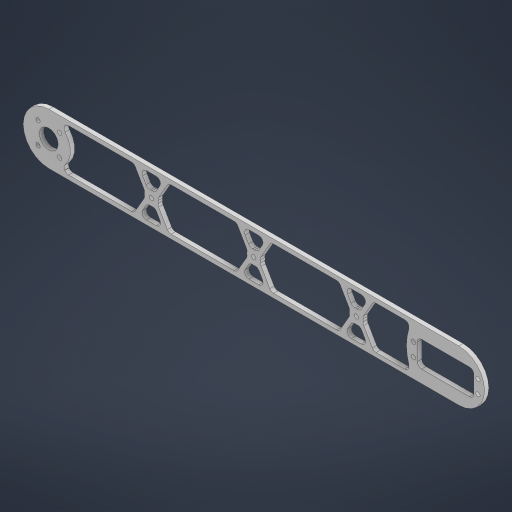
# Autodesk Inventor part: Arm2ndLink
Saved by Autodesk Inventor 2023 (Build 270158000, 158)
## iProperties
Created: 2023-12-24
Part Number: Arm2ndLink
Material: Generic
Document SubType Name: Modeling
Designer: kelle
Density: 1 g/cm^3
Appearance: Default
Author: kelle
Autodesk Inventor part; units mm, degrees
ref_plane "YZ Plane" through (0, 0, 0) normal (1, 0, 0) x (0, 1, 0)
ref_plane "XZ Plane" through (0, 0, 0) normal (0, 1, 0) x (-1, 0, 0)
ref_plane "XY Plane" through (0, 0, 0) normal (0, 0, 1) x (1, 0, 0)
sketch "Sketch1" plane through (0, 0, 0) normal (0, 0, 1) x (1, 0, 0)
  line L0 (152.4, 0) -> (-152.4, 0) construction
  line L1 (152.4, 19.05) -> (-152.4, 19.05)
  line L2 (-152.4, -19.05) -> (152.4, -19.05)
  arc A0 (152.4, -19.05) -> (152.4, 19.05) centre (152.4, 0) ccw
  arc A1 (-152.4, 19.05) -> (-152.4, -19.05) centre (-152.4, 0) ccw
  circle A2 centre (-152.4, 0) radius 7
  line L3 (-160.4, -8) -> (-144.4, -8) construction
  line L4 (-144.4, -8) -> (-144.4, 8) construction
  line L5 (-144.4, 8) -> (-160.4, 8) construction
  line L6 (-160.4, 8) -> (-160.4, -8) construction
  line L7 (-160.4, -8) -> (-144.4, 8) construction
  line L8 (-144.4, -8) -> (-160.4, 8) construction
  circle A3 centre (-160.4, 8) radius 1.5875
  circle A4 centre (-144.4, 8) radius 1.5875
  circle A5 centre (-160.4, -8) radius 1.5875
  circle A6 centre (-144.4, -8) radius 1.5875
  circle A7 centre (0, 0) radius 2
  circle A8 centre (-76.2, 0) radius 2
  circle A9 centre (76.2, 0) radius 2
  circle A10 centre (0, 0) radius 2
  circle A11 centre (152.4, 0) radius 3
  line L9 (152.4, 0) -> (166.6, 0) construction
  line L10 (166.6, 0) -> (166.6, 4.95) construction
  circle A12 centre (166.6, 4.95) radius 1.5875
  circle A13 centre (118.6, 4.95) radius 1.5875
  circle A14 centre (166.6, -4.95) radius 1.5875
  circle A15 centre (118.6, -4.95) radius 1.5875
  line L11 (166.6, 4.95) -> (163.6, 4.95) construction
  line L12 (163.6, 9.525) -> (121.6, 9.525)
  line L13 (121.6, 9.525) -> (121.6, -9.525)
  line L14 (163.6, -9.525) -> (163.6, 9.525)
  line L15 (121.6, -9.525) -> (163.6, -9.525)
  dimension "d0" = 152.4
  dimension "d1" = 38.1
  dimension "d2" = 14
  dimension "d3" = 16
  dimension "d4" = 16
  dimension "d5" = 3.175
  dimension "d8" = 16
  dimension "d11" = 16
  dimension "d14" = 4
  dimension "d17" = 76.2
  dimension "d20" = 76.2
  dimension "d23" = 6
  dimension "d24" = 14.2
  dimension "d25" = 4.95
  dimension "d27" = 3.175
  dimension "d31" = 48
  dimension "d34" = 9.9
  dimension "d37" = 3
  dimension "d38" = 42
  dimension "d39" = 9.525
  dimension "d40" = 19.05
  dimension "d41" = 42
  constraints: 34 end point, 16 centre point, 9 horizontal, 5 coincident, 4 point on circle, 4 tangent, 4 vertical, 3 midpoint, 3 parallel, 1 perpendicular, 18 other
  measures "d0" distance of point (0, 0) L0.end
  measures "d1" diameter of A1
  measures "d2" diameter of A2
  measures "d3" distance of L3.start L3.end
  measures "d4" distance of L4.end L3.end
  measures "d5" diameter of A3
  measures "d8" distance of A3.centre A4.centre
  measures "d11" distance of A3.centre A5.centre
  measures "d14" diameter of A7
  measures "d17" distance of A7.centre A8.centre
  measures "d20" distance of A7.centre A9.centre
  measures "d23" diameter of A11
  measures "d24" distance of L9.start L9.end
  measures "d25" distance of L9.end L10.end
  measures "d27" diameter of A12
  measures "d31" distance of L11.start A13.centre
  measures "d34" distance of L11.start A14.centre
  measures "d37" distance of L11.start L11.end
  measures "d38" distance of L12.start L12.end
  measures "d39" distance between parallel lines of L12 L0
  measures "d40" distance of L12.end L13.end
  measures "d41" distance of L13.end L14.start
extrude "Extrusion1" add sketch "Sketch1" along normal blind 3.175 contours A0 L2 A1 L1
sketch "Sketch2" plane through (0, 0, 3.175) normal (0, 0, 1) x (1, 0, 0)
  arc A0 (-152.4, 19.05) -> (-152.4, -19.05) centre (-152.4, 0) ccw projected
  line L0 (-152.4, -19.05) -> (152.4, -19.05) projected
  arc A1 (152.4, -19.05) -> (152.4, 19.05) centre (152.4, 0) ccw projected
  line L1 (152.4, 19.05) -> (-152.4, 19.05) projected
  circle A2 centre (0, 0) radius 2 projected
  circle A3 centre (-76.2, 0) radius 2 projected
  circle A4 centre (76.2, 0) radius 2 projected
  circle A5 centre (118.6, 4.95) radius 1.5875 projected
  circle A6 centre (118.6, -4.95) radius 1.5875 projected
  circle A7 centre (166.6, -4.95) radius 1.5875 projected
  circle A8 centre (166.6, 4.95) radius 1.5875 projected
  circle A9 centre (-144.4, -8) radius 1.5875 projected
  circle A10 centre (-160.4, -8) radius 1.5875 projected
  circle A11 centre (-144.4, 8) radius 1.5875 projected
  circle A12 centre (-160.4, 8) radius 1.5875 projected
  circle A13 centre (-152.4, 0) radius 7 projected
  line L2 (-152.4, 0) -> (-114.3, 0) construction
  arc A14 (-152.4, 15.875) -> (-152.4, -15.875) centre (-152.4, 0) ccw
  line L3 (-152.4, -15.875) -> (152.4, -15.875)
  arc A15 (152.4, -15.875) -> (152.4, 15.875) centre (152.4, 0) ccw
  line L4 (152.4, 15.875) -> (-152.4, 15.875)
  circle A16 centre (-76.2, 0) radius 5.175
  circle A17 centre (0, 0) radius 5.175
  circle A18 centre (76.2, 0) radius 5.175
  circle A19 centre (-152.4, 0) radius 12.9012 construction
  circle A20 centre (152.4, 0) radius 35.748 construction
  circle A21 centre (152.4, 0) radius 38.923
  circle A22 centre (-152.4, 0) radius 16.0762
  line L5 (-152.4, 0) -> (-133.35, 32.9956)
  line L6 (-133.35, 32.9956) -> (-95.25, 32.9956) construction
  line L7 (-95.25, 32.9956) -> (-76.2, 0)
  line L8 (-76.2, 0) -> (-95.25, -32.9956)
  line L9 (-95.25, -32.9956) -> (-133.35, -32.9956) construction
  line L10 (-133.35, -32.9956) -> (-152.4, 0)
  line L11 (0, 19.05) -> (0, -19.05) construction
  line L12 (-76.2, 19.05) -> (-76.2, -19.05) construction
  line L13 (-97.0831, 29.8206) -> (-131.5169, 29.8206)
  line L14 (-131.5169, 29.8206) -> (-148.7338, 0)
  line L15 (-148.7338, 0) -> (-131.5169, -29.8206)
  line L16 (-131.5169, -29.8206) -> (-97.0831, -29.8206)
  line L17 (-97.0831, -29.8206) -> (-79.8662, 0)
  line L18 (-79.8662, 0) -> (-97.0831, 29.8206)
  line L19 (-20.8831, 29.8206) -> (-3.6662, 0)
  line L20 (-3.6662, 0) -> (-20.8831, -29.8206)
  line L21 (-55.3169, -29.8206) -> (-72.5338, 0)
  line L22 (-72.5338, 0) -> (-55.3169, 29.8206)
  line L23 (131.5169, 29.8206) -> (148.7338, 0)
  line L24 (148.7338, 0) -> (131.5169, -29.8206)
  line L25 (97.0831, -29.8206) -> (79.8662, 0)
  line L26 (79.8662, 0) -> (97.0831, 29.8206)
  line L27 (20.8831, 29.8206) -> (3.6662, 0)
  line L28 (72.5338, 0) -> (55.3169, 29.8206)
  line L29 (55.3169, -29.8206) -> (72.5338, 0)
  line L30 (3.6662, 0) -> (20.8831, -29.8206)
  line L31 (0, 0) -> (-19.05, 32.9956)
  line L32 (-57.15, 32.9956) -> (-76.2, 0)
  line L33 (-76.2, 0) -> (-57.15, -32.9956)
  line L34 (-19.05, -32.9956) -> (0, 0)
  line L35 (152.4, 0) -> (133.35, 32.9956)
  line L36 (95.25, 32.9956) -> (76.2, 0)
  line L37 (76.2, 0) -> (95.25, -32.9956)
  line L38 (133.35, -32.9956) -> (152.4, 0)
  line L39 (19.05, -32.9956) -> (0, 0)
  line L40 (0, 0) -> (19.05, 32.9956)
  line L41 (57.15, 32.9956) -> (76.2, 0)
  line L42 (76.2, 0) -> (57.15, -32.9956)
  point P0 (73.6125, -4.4817)
  point P1 (67.0346, -15.875)
  point P2 (85.3654, -15.875)
  point P3 (78.7875, -4.4817)
  point P4 (80.9929, -1.9516)
  point P5 (89.0316, -15.875)
  point P6 (116.8615, -15.875)
  point P7 (116.8615, 15.875)
  point P8 (89.0316, 15.875)
  point P9 (80.9929, 1.9516)
  point P10 (67.0346, 15.875)
  point P11 (73.6125, 4.4817)
  point P12 (78.7875, 4.4817)
  point P13 (85.3654, 15.875)
  point P14 (9.1654, -15.875)
  point P15 (2.5875, -4.4817)
  point P16 (-2.5875, -4.4817)
  point P17 (-9.1654, -15.875)
  point P18 (4.7929, -1.9516)
  point P19 (12.8316, -15.875)
  point P20 (63.3684, -15.875)
  point P21 (71.4071, -1.9516)
  point P22 (71.4071, 1.9516)
  point P23 (63.3684, 15.875)
  point P24 (12.8316, 15.875)
  point P25 (4.7929, 1.9516)
  point P26 (2.5875, 4.4817)
  point P27 (9.1654, 15.875)
  point P28 (-9.1654, 15.875)
  point P29 (-2.5875, 4.4817)
  point P30 (-67.0346, -15.875)
  point P31 (-73.6125, -4.4817)
  point P32 (-78.7875, -4.4817)
  point P33 (-85.3654, -15.875)
  point P34 (-12.8316, -15.875)
  point P35 (-4.7929, -1.9516)
  point P36 (-4.7929, 1.9516)
  point P37 (-12.8316, 15.875)
  point P38 (-63.3684, 15.875)
  point P39 (-71.4071, 1.9516)
  point P40 (-71.4071, -1.9516)
  point P41 (-63.3684, -15.875)
  point P42 (-73.6125, 4.4817)
  point P43 (-67.0346, 15.875)
  point P44 (-85.3654, 15.875)
  point P45 (-78.7875, 4.4817)
  point P46 (-80.9929, 1.9516)
  point P47 (-89.0316, 15.875)
  point P48 (-139.5684, 15.875)
  point P49 (-141.7706, 12.0607)
  point P50 (-141.7706, -12.0607)
  point P51 (-139.5684, -15.875)
  point P52 (-89.0316, -15.875)
  point P53 (-80.9929, -1.9516)
  dimension "d44" = 38.1
  dimension "d45" = 3.175
  dimension "d46" = 3.175
  dimension "d47" = 3.175
  dimension "d48" = 3.175
  dimension "d49" = 3.175
  dimension "d50" = 3.175
  dimension "d51" = 3.175
  constraints: 82 end point, 33 symmetric about line, 9 centre point, 4 point on circle, 3 coincident, 2 midpoint, 2 point on line, 2 tangent, 1 horizontal, 1 perpendicular, 21 other
  measures "d44" distance of L2.start L2.end
  measures "d45" distance between parallel lines of L1 L4
  measures "d46" radial gap between concentric circles of A3 A16
  measures "d47" radial gap between concentric circles of A2 A17
  measures "d48" radial gap between concentric circles of A4 A18
  measures "d49" radial gap between concentric circles of A20 A21
  measures "d50" radial gap between concentric circles of A19 A22
  measures "d51" distance between parallel lines of L6 L13
extrude "Extrusion2" cut sketch "Sketch2" against normal through all contours L4 L18 A16 L17 L3 L15 A22 L14 | L4 L32 A16 L7 | L8 A16 L33 L3 | L4 L19 A17 L20 L3 L21 A16 L22 | L4 L40 A17 L31 | L34 A17 L39 L3 | L4 L28 A18 L29 L3 L30 A17 L27 | L4 L36 A18 L41 | L42 A18 L37 L3 | L4 A21 L3 L25 A18 L26
fillet "Fillet1" radius 3.175 58 edges at (-73.6125, -4.4817, 1.5875) (-67.0346, -15.875, 1.5875) (-78.7875, -4.4817, 1.5875) (-85.3654, -15.875, 1.5875) (2.5875, -4.4817, 1.5875) (9.1654, -15.875, 1.5875) (-2.5875, -4.4817, 1.5875) (-9.1654, -15.875, 1.5875) (67.0346, -15.875, 1.5875) (73.6125, -4.4817, 1.5875) (85.3654, -15.875, 1.5875) (78.7875, -4.4817, 1.5875) (-89.0316, 15.875, 1.5875) (-80.9929, 1.9516, 1.5875) (-139.5684, 15.875, 1.5875) (-141.7706, 12.0607, 1.5875) (-141.7706, -12.0607, 1.5875) (-139.5684, -15.875, 1.5875) (-89.0316, -15.875, 1.5875) (-80.9929, -1.9516, 1.5875) (-4.7929, -1.9516, 1.5875) (-12.8316, -15.875, 1.5875) (-4.7929, 1.9516, 1.5875) (-12.8316, 15.875, 1.5875) (-63.3684, 15.875, 1.5875) (-71.4071, 1.9516, 1.5875) (-71.4071, -1.9516, 1.5875) (-63.3684, -15.875, 1.5875) (-67.0346, 15.875, 1.5875) (-73.6125, 4.4817, 1.5875) (-85.3654, 15.875, 1.5875) (-78.7875, 4.4817, 1.5875) (9.1654, 15.875, 1.5875) (2.5875, 4.4817, 1.5875) (-9.1654, 15.875, 1.5875) (-2.5875, 4.4817, 1.5875) (12.8316, -15.875, 1.5875) (4.7929, -1.9516, 1.5875) (63.3684, -15.875, 1.5875) (71.4071, -1.9516, 1.5875) (71.4071, 1.9516, 1.5875) (63.3684, 15.875, 1.5875) (12.8316, 15.875, 1.5875) (4.7929, 1.9516, 1.5875) (89.0316, -15.875, 1.5875) (80.9929, -1.9516, 1.5875) (116.8615, -15.875, 1.5875) (116.8615, 15.875, 1.5875) (89.0316, 15.875, 1.5875) (80.9929, 1.9516, 1.5875) (163.6, 9.525, 1.5875) (163.6, -9.525, 1.5875) (121.6, 9.525, 1.5875) (121.6, -9.525, 1.5875) (73.6125, 4.4817, 1.5875) (67.0346, 15.875, 1.5875) (78.7875, 4.4817, 1.5875) (85.3654, 15.875, 1.5875)
sketch "Sketch3" plane through (0, 0, 3.175) normal (0, 0, 1) x (1, 0, 0)
  line L0 (-11.9151, 14.2875) -> (-5.4607, 3.1082) projected
  arc A0 (-5.0885, 0.9425) -> (-5.4607, 3.1082) centre (-8.2103, 1.5207) ccw projected
  arc A1 (-5.0885, 0.9425) -> (-5.0885, -0.9425) centre (0, 0) ccw projected
  arc A2 (-5.4607, -3.1082) -> (-5.0885, -0.9425) centre (-8.2103, -1.5207) ccw projected
  line L1 (-5.4607, -3.1082) -> (-11.9151, -14.2875) projected
  arc A3 (-14.6647, -15.875) -> (-11.9151, -14.2875) centre (-14.6647, -12.7) ccw projected
  line L2 (-14.6647, -15.875) -> (-61.5353, -15.875) projected
  arc A4 (-64.2849, -14.2875) -> (-61.5353, -15.875) centre (-61.5353, -12.7) ccw projected
  line L3 (-64.2849, -14.2875) -> (-70.7393, -3.1082) projected
  arc A5 (-71.1115, -0.9425) -> (-70.7393, -3.1082) centre (-67.9897, -1.5207) ccw projected
  arc A6 (-71.1115, -0.9425) -> (-71.1115, 0.9425) centre (-76.2, 0) ccw projected
  arc A7 (-70.7393, 3.1082) -> (-71.1115, 0.9425) centre (-67.9897, 1.5207) ccw projected
  line L4 (-70.7393, 3.1082) -> (-64.2849, 14.2875) projected
  arc A8 (-61.5353, 15.875) -> (-64.2849, 14.2875) centre (-61.5353, 12.7) ccw projected
  line L5 (-61.5353, 15.875) -> (-14.6647, 15.875) projected
  arc A9 (-11.9151, 14.2875) -> (-14.6647, 15.875) centre (-14.6647, 12.7) ccw projected
  line L6 (-6.4158, -11.1125) -> (-3.8614, -6.6882) projected
  arc A10 (-0.689, -5.1289) -> (-3.8614, -6.6882) centre (-1.1118, -8.2757) ccw projected
  arc A11 (-0.689, -5.1289) -> (0.689, -5.1289) centre (0, 0) ccw projected
  arc A12 (3.8614, -6.6882) -> (0.689, -5.1289) centre (1.1118, -8.2757) ccw projected
  line L7 (3.8614, -6.6882) -> (6.4158, -11.1125) projected
  arc A13 (3.6662, -15.875) -> (6.4158, -11.1125) centre (3.6662, -12.7) ccw projected
  line L8 (3.6662, -15.875) -> (-3.6662, -15.875) projected
  arc A14 (-6.4158, -11.1125) -> (-3.6662, -15.875) centre (-3.6662, -12.7) ccw projected
  line L9 (80.0614, -6.6882) -> (82.6158, -11.1125) projected
  arc A15 (79.8662, -15.875) -> (82.6158, -11.1125) centre (79.8662, -12.7) ccw projected
  line L10 (79.8662, -15.875) -> (72.5338, -15.875) projected
  arc A16 (69.7842, -11.1125) -> (72.5338, -15.875) centre (72.5338, -12.7) ccw projected
  line L11 (69.7842, -11.1125) -> (72.3386, -6.6882) projected
  arc A17 (75.511, -5.1289) -> (72.3386, -6.6882) centre (75.0882, -8.2757) ccw projected
  arc A18 (75.511, -5.1289) -> (76.889, -5.1289) centre (76.2, 0) ccw projected
  arc A19 (80.0614, -6.6882) -> (76.889, -5.1289) centre (77.3118, -8.2757) ccw projected
  line L12 (70.7393, -3.1082) -> (64.2849, -14.2875) projected
  arc A20 (61.5353, -15.875) -> (64.2849, -14.2875) centre (61.5353, -12.7) ccw projected
  line L13 (61.5353, -15.875) -> (14.6647, -15.875) projected
  arc A21 (11.9151, -14.2875) -> (14.6647, -15.875) centre (14.6647, -12.7) ccw projected
  line L14 (11.9151, -14.2875) -> (5.4607, -3.1082) projected
  arc A22 (5.0885, -0.9425) -> (5.4607, -3.1082) centre (8.2103, -1.5207) ccw projected
  arc A23 (5.0885, -0.9425) -> (5.0885, 0.9425) centre (0, 0) ccw projected
  arc A24 (5.4607, 3.1082) -> (5.0885, 0.9425) centre (8.2103, 1.5207) ccw projected
  line L15 (5.4607, 3.1082) -> (11.9151, 14.2875) projected
  arc A25 (14.6647, 15.875) -> (11.9151, 14.2875) centre (14.6647, 12.7) ccw projected
  line L16 (14.6647, 15.875) -> (61.5353, 15.875) projected
  arc A26 (64.2849, 14.2875) -> (61.5353, 15.875) centre (61.5353, 12.7) ccw projected
  line L17 (64.2849, 14.2875) -> (70.7393, 3.1082) projected
  arc A27 (71.1115, 0.9425) -> (70.7393, 3.1082) centre (67.9897, 1.5207) ccw projected
  arc A28 (71.1115, 0.9425) -> (71.1115, -0.9425) centre (76.2, 0) ccw projected
  arc A29 (70.7393, -3.1082) -> (71.1115, -0.9425) centre (67.9897, -1.5207) ccw projected
  line L18 (-80.0614, 6.6882) -> (-82.6158, 11.1125) projected
  arc A30 (-79.8662, 15.875) -> (-82.6158, 11.1125) centre (-79.8662, 12.7) ccw projected
  line L19 (-79.8662, 15.875) -> (-72.5338, 15.875) projected
  arc A31 (-69.7842, 11.1125) -> (-72.5338, 15.875) centre (-72.5338, 12.7) ccw projected
  line L20 (-69.7842, 11.1125) -> (-72.3386, 6.6882) projected
  arc A32 (-75.511, 5.1289) -> (-72.3386, 6.6882) centre (-75.0882, 8.2757) ccw projected
  arc A33 (-75.511, 5.1289) -> (-76.889, 5.1289) centre (-76.2, 0) ccw projected
  arc A34 (-80.0614, 6.6882) -> (-76.889, 5.1289) centre (-77.3118, 8.2757) ccw projected
  line L21 (-82.6158, -11.1125) -> (-80.0614, -6.6882) projected
  arc A35 (-76.889, -5.1289) -> (-80.0614, -6.6882) centre (-77.3118, -8.2757) ccw projected
  arc A36 (-76.889, -5.1289) -> (-75.511, -5.1289) centre (-76.2, 0) ccw projected
  arc A37 (-72.3386, -6.6882) -> (-75.511, -5.1289) centre (-75.0882, -8.2757) ccw projected
  line L22 (-72.3386, -6.6882) -> (-69.7842, -11.1125) projected
  arc A38 (-72.5338, -15.875) -> (-69.7842, -11.1125) centre (-72.5338, -12.7) ccw projected
  line L23 (-72.5338, -15.875) -> (-79.8662, -15.875) projected
  arc A39 (-82.6158, -11.1125) -> (-79.8662, -15.875) centre (-79.8662, -12.7) ccw projected
  line L24 (82.6158, 11.1125) -> (80.0614, 6.6882) projected
  arc A40 (76.889, 5.1289) -> (80.0614, 6.6882) centre (77.3118, 8.2757) ccw projected
  arc A41 (76.889, 5.1289) -> (75.511, 5.1289) centre (76.2, 0) ccw projected
  arc A42 (72.3386, 6.6882) -> (75.511, 5.1289) centre (75.0882, 8.2757) ccw projected
  line L25 (72.3386, 6.6882) -> (69.7842, 11.1125) projected
  arc A43 (72.5338, 15.875) -> (69.7842, 11.1125) centre (72.5338, 12.7) ccw projected
  line L26 (72.5338, 15.875) -> (79.8662, 15.875) projected
  arc A44 (82.6158, 11.1125) -> (79.8662, 15.875) centre (79.8662, 12.7) ccw projected
  arc A45 (115.2904, 11.7422) -> (115.2904, -11.7422) centre (152.4, 0) ccw projected
  arc A46 (112.2633, -15.875) -> (115.2904, -11.7422) centre (112.2633, -12.7) ccw projected
  line L27 (112.2633, -15.875) -> (90.8647, -15.875) projected
  arc A47 (88.1151, -14.2875) -> (90.8647, -15.875) centre (90.8647, -12.7) ccw projected
  line L28 (88.1151, -14.2875) -> (81.6607, -3.1082) projected
  arc A48 (81.2885, -0.9425) -> (81.6607, -3.1082) centre (84.4103, -1.5207) ccw projected
  arc A49 (81.2885, -0.9425) -> (81.2885, 0.9425) centre (76.2, 0) ccw projected
  arc A50 (81.6607, 3.1082) -> (81.2885, 0.9425) centre (84.4103, 1.5207) ccw projected
  line L29 (81.6607, 3.1082) -> (88.1151, 14.2875) projected
  arc A51 (90.8647, 15.875) -> (88.1151, 14.2875) centre (90.8647, 12.7) ccw projected
  line L30 (90.8647, 15.875) -> (112.2633, 15.875) projected
  arc A52 (115.2904, 11.7422) -> (112.2633, 15.875) centre (112.2633, 12.7) ccw projected
  line L31 (-3.8614, 6.6882) -> (-6.4158, 11.1125) projected
  arc A53 (-3.6662, 15.875) -> (-6.4158, 11.1125) centre (-3.6662, 12.7) ccw projected
  line L32 (-3.6662, 15.875) -> (3.6662, 15.875) projected
  arc A54 (6.4158, 11.1125) -> (3.6662, 15.875) centre (3.6662, 12.7) ccw projected
  line L33 (6.4158, 11.1125) -> (3.8614, 6.6882) projected
  arc A55 (0.689, 5.1289) -> (3.8614, 6.6882) centre (1.1118, 8.2757) ccw projected
  arc A56 (0.689, 5.1289) -> (-0.689, 5.1289) centre (0, 0) ccw projected
  arc A57 (-3.8614, 6.6882) -> (-0.689, 5.1289) centre (-1.1118, 8.2757) ccw projected
  line L34 (-140.5635, 14.1515) -> (-140.4849, 14.2875) projected
  arc A58 (-137.7353, 15.875) -> (-140.4849, 14.2875) centre (-137.7353, 12.7) ccw projected
  line L35 (-137.7353, 15.875) -> (-90.8647, 15.875) projected
  arc A59 (-88.1151, 14.2875) -> (-90.8647, 15.875) centre (-90.8647, 12.7) ccw projected
  line L36 (-88.1151, 14.2875) -> (-81.6607, 3.1082) projected
  arc A60 (-81.2885, 0.9425) -> (-81.6607, 3.1082) centre (-84.4103, 1.5207) ccw projected
  arc A61 (-81.2885, 0.9425) -> (-81.2885, -0.9425) centre (-76.2, 0) ccw projected
  arc A62 (-81.6607, -3.1082) -> (-81.2885, -0.9425) centre (-84.4103, -1.5207) ccw projected
  line L37 (-81.6607, -3.1082) -> (-88.1151, -14.2875) projected
  arc A63 (-90.8647, -15.875) -> (-88.1151, -14.2875) centre (-90.8647, -12.7) ccw projected
  line L38 (-90.8647, -15.875) -> (-137.7353, -15.875) projected
  arc A64 (-140.4849, -14.2875) -> (-137.7353, -15.875) centre (-137.7353, -12.7) ccw projected
  line L39 (-140.4849, -14.2875) -> (-140.5635, -14.1515) projected
  arc A65 (-140.2195, -10.4919) -> (-140.5635, -14.1515) centre (-137.8138, -12.564) ccw projected
  arc A66 (-140.2195, -10.4919) -> (-140.2195, 10.4919) centre (-152.4, 0) ccw projected
  arc A67 (-140.5635, 14.1515) -> (-140.2195, 10.4919) centre (-137.8138, 12.564) ccw projected
  arc A68 (-152.4, 19.05) -> (-152.4, -19.05) centre (-152.4, 0) ccw projected
  line L40 (-152.4, -19.05) -> (152.4, -19.05) projected
  arc A69 (152.4, -19.05) -> (152.4, 19.05) centre (152.4, 0) ccw projected
  line L41 (152.4, 19.05) -> (-152.4, 19.05) projected
  circle A70 centre (0, 0) radius 2 projected
  circle A71 centre (-76.2, 0) radius 2 projected
  circle A72 centre (76.2, 0) radius 2 projected
  circle A73 centre (118.6, 4.95) radius 1.5875 projected
  circle A74 centre (118.6, -4.95) radius 1.5875 projected
  circle A75 centre (166.6, -4.95) radius 1.5875 projected
  circle A76 centre (166.6, 4.95) radius 1.5875 projected
  circle A77 centre (-144.4, -8) radius 1.5875 projected
  circle A78 centre (-160.4, -8) radius 1.5875 projected
  circle A79 centre (-144.4, 8) radius 1.5875 projected
  circle A80 centre (-160.4, 8) radius 1.5875 projected
  circle A81 centre (-152.4, 0) radius 7 projected
  circle A82 centre (-76.2, 0) radius 2 projected
  circle A83 centre (-76.2, 0) radius 1.5875
  circle A84 centre (0, 0) radius 1.5875
  circle A85 centre (76.2, 0) radius 2 projected
  circle A86 centre (76.2, 0) radius 1.5875
  dimension "d55" = 3.175
  dimension "d56" = 3.175
  dimension "d57" = 3.175
  constraints: 3 centre point, 3 coincident
  measures "d55" diameter of A83
  measures "d56" diameter of A84
  measures "d57" diameter of A86
extrude "Extrusion3" add sketch "Sketch3" against normal blind 3.175 contours A70 | A71 | A72
body "Solid1"
